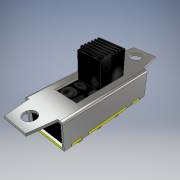
# Autodesk Inventor part: Switch-T220
Saved by Autodesk Inventor 2018 (Build 220112000, 112)
## iProperties
Created: 2021-02-15
Part Number: Switch-T220
Material: Všeobecné
Document SubType Name: Modeling
Designer: Jozko Mrkvicka
Density: 1 g/cm^3
Appearance: Výchozí
Author: Jozko Mrkvicka
Autodesk Inventor part; units mm, degrees
ref_plane "YZ Plane" through (0, 0, 0) normal (1, 0, 0) x (0, 1, 0)
ref_plane "XZ Plane" through (0, 0, 0) normal (0, 1, 0) x (-1, 0, 0)
sketch "Náčrt1" plane through (0, 0, 0) normal (0, 1, 0) x (-1, 0, 0)
  line L0 (-3.175, 18.0975) -> (3.175, 18.0975)
  line L1 (5.3975, 12.065) -> (5.3975, -12.065)
  line L2 (3.175, -18.0975) -> (-3.175, -18.0975)
  line L3 (-5.3975, -12.065) -> (-5.3975, 12.065)
  line L4 (3.175, 18.0975) -> (4.1275, 12.065)
  line L5 (-4.1275, 12.065) -> (-3.175, 18.0975)
  line L6 (-4.1275, -12.065) -> (-3.175, -18.0975)
  line L7 (4.1275, -12.065) -> (3.175, -18.0975)
  circle A0 centre (0, 14.9225) radius 1.5875
  circle A1 centre (0, -14.9225) radius 1.5875
  line L8 (-5.3975, 12.065) -> (-4.1275, 12.065)
  line L9 (4.1275, 12.065) -> (5.3975, 12.065)
  line L10 (5.3975, -12.065) -> (4.1275, -12.065)
  line L11 (-4.1275, -12.065) -> (-5.3975, -12.065)
  line L12 (-3.175, 6.6675) -> (3.175, 6.6675)
  line L13 (3.175, 6.6675) -> (3.175, -6.6675)
  line L14 (3.175, -6.6675) -> (-3.175, -6.6675)
  line L15 (-3.175, -6.6675) -> (-3.175, 6.6675)
  line L16 (-3.175, 6.6675) -> (3.175, -6.6675) construction
  line L17 (3.175, 6.6675) -> (-3.175, -6.6675) construction
  point P0 (0, 0)
  dimension "d7" = 6.35
  dimension "d8" = 13.335
  constraints: 36 end point, 8 parallel, 4 horizontal, 2 centre point, 2 midpoint, 2 perpendicular
  measures "d7" distance of L13.end L14.end
  measures "d8" distance of L12.end L13.end
extrude "Vysunutí1" add sketch "Náčrt1" along normal blind 0.635
sketch "Náčrt2" plane through (0, 0, 0) normal (0, -1, 0) x (1, 0, 0)
  line L0 (5.3975, 12.065) -> (4.1275, 12.065) projected
  line L1 (-5.3975, -12.065) -> (-5.3975, 12.065) projected
  line L2 (5.3975, 12.065) -> (-5.3975, 12.065)
  line L3 (-5.3975, 12.065) -> (-5.3975, -12.065)
  line L4 (-5.3975, -12.065) -> (5.3975, -12.065)
  line L5 (5.3975, -12.065) -> (5.3975, 12.065)
  constraints: 8 end point, 2 parallel, 1 horizontal, 1 perpendicular
extrude "Vysunutí2" add sketch "Náčrt2" along normal blind 6.35
sketch "Náčrt3" plane through (0, 0, 0) normal (0, 1, 0) x (1, 0, 0)
  line L0 (3.175, 6.6675) -> (3.175, -6.6675) projected
  line L1 (-3.175, -6.6675) -> (3.175, -6.6675)
  line L2 (3.175, -6.6675) -> (3.175, 0.3175)
  line L3 (3.175, 0.3175) -> (-3.175, 0.3175)
  line L4 (-3.175, 0.3175) -> (-3.175, -6.6675)
  point P0 (0, 0)
  dimension "d13" = 6.985
  constraints: 8 end point, 2 parallel, 1 horizontal, 1 perpendicular, 1 point on line
  measures "d13" distance of L2.end L1.end
extrude "Vysunutí3" add sketch "Náčrt3" along normal blind 6.985
sketch "Náčrt4" plane through (3.175, 0.635, -0.3175) normal (1, 0, 0) x (0, 0, -1)
  line L0 (-6.985, 6.35) -> (0, 6.35) projected
  line L1 (-6.223, 6.35) -> (-5.588, 6.35)
  line L2 (-5.588, 6.35) -> (-5.588, 6.6675)
  line L3 (-6.223, 6.6675) -> (-6.223, 6.35)
  arc A0 (-5.588, 6.6675) -> (-6.223, 6.6675) centre (-5.9055, 6.6675) ccw
  line L4 (-5.2705, 6.35) -> (-4.6355, 6.35)
  line L5 (-4.6355, 6.35) -> (-4.6355, 6.6675)
  line L6 (-5.2705, 6.6675) -> (-5.2705, 6.35)
  arc A1 (-4.6355, 6.6675) -> (-5.2705, 6.6675) centre (-4.953, 6.6675) ccw
  line L7 (-4.318, 6.35) -> (-3.683, 6.35)
  line L8 (-3.683, 6.35) -> (-3.683, 6.6675)
  line L9 (-4.318, 6.6675) -> (-4.318, 6.35)
  arc A2 (-3.683, 6.6675) -> (-4.318, 6.6675) centre (-4.0005, 6.6675) ccw
  line L10 (-3.3655, 6.35) -> (-2.7305, 6.35)
  line L11 (-2.7305, 6.35) -> (-2.7305, 6.6675)
  line L12 (-3.3655, 6.6675) -> (-3.3655, 6.35)
  arc A3 (-2.7305, 6.6675) -> (-3.3655, 6.6675) centre (-3.048, 6.6675) ccw
  line L13 (-2.413, 6.35) -> (-1.778, 6.35)
  line L14 (-1.778, 6.35) -> (-1.778, 6.6675)
  line L15 (-2.413, 6.6675) -> (-2.413, 6.35)
  arc A4 (-1.778, 6.6675) -> (-2.413, 6.6675) centre (-2.0955, 6.6675) ccw
  line L16 (-1.4605, 6.35) -> (-0.8255, 6.35)
  line L17 (-0.8255, 6.35) -> (-0.8255, 6.6675)
  line L18 (-1.4605, 6.6675) -> (-1.4605, 6.35)
  arc A5 (-0.8255, 6.6675) -> (-1.4605, 6.6675) centre (-1.143, 6.6675) ccw
  point P0 (-0.3175, -0.635)
  dimension "d28" = 0.9525
  constraints: 36 end point, 12 point on circle, 6 centre point, 2 horizontal, 1 parallel, 1 perpendicular, 1 point on line, 45 other
  measures "d28" distance of L1.start L4.start
extrude "Vysunutí4" add sketch "Náčrt4" against normal up to surface (6.35 mm away)
fillet "Zaoblení1" radius 0.635 2 edges at (5.3975, 0.635, 0) (-5.3975, 0.635, 0)
sketch "Náčrt5" plane through (0, -6.35, 0) normal (0, -1, 0) x (1, 0, 0)
  line L0 (5.3975, 12.065) -> (4.7625, 12.065)
  line L1 (4.7625, 12.065) -> (4.7625, 10.16)
  line L2 (4.7625, 10.16) -> (5.3975, 10.16)
  line L3 (5.3975, 10.16) -> (5.3975, 12.065)
  line L4 (5.3975, -12.065) -> (4.7625, -12.065)
  line L5 (4.7625, -12.065) -> (4.7625, -10.16)
  line L6 (4.7625, -10.16) -> (5.3975, -10.16)
  line L7 (5.3975, -10.16) -> (5.3975, -12.065)
  line L8 (-5.3975, -12.065) -> (-4.7625, -12.065)
  line L9 (-4.7625, -12.065) -> (-4.7625, -10.16)
  line L10 (-4.7625, -10.16) -> (-5.3975, -10.16)
  line L11 (-5.3975, -10.16) -> (-5.3975, -12.065)
  line L12 (-5.3975, 12.065) -> (-4.7625, 12.065)
  line L13 (-4.7625, 12.065) -> (-4.7625, 10.16)
  line L14 (-4.7625, 10.16) -> (-5.3975, 10.16)
  line L15 (-5.3975, 10.16) -> (-5.3975, 12.065)
  line L16 (4.7625, -7.62) -> (5.3975, -7.62)
  line L17 (5.3975, -7.62) -> (5.3975, -5.715)
  line L18 (5.3975, -5.715) -> (4.7625, -5.715)
  line L19 (4.7625, -5.715) -> (4.7625, -7.62)
  line L20 (-4.7625, 7.62) -> (-5.3975, 7.62)
  line L21 (-5.3975, 7.62) -> (-5.3975, 5.715)
  line L22 (-5.3975, 5.715) -> (-4.7625, 5.715)
  line L23 (-4.7625, 5.715) -> (-4.7625, 7.62)
  line L24 (4.7625, 7.62) -> (5.3975, 7.62)
  line L25 (5.3975, 7.62) -> (5.3975, 5.715)
  line L26 (5.3975, 5.715) -> (4.7625, 5.715)
  line L27 (4.7625, 5.715) -> (4.7625, 7.62)
  line L28 (-4.7625, -7.62) -> (-5.3975, -7.62)
  line L29 (-5.3975, -7.62) -> (-5.3975, -5.715)
  line L30 (-5.3975, -5.715) -> (-4.7625, -5.715)
  line L31 (-4.7625, -5.715) -> (-4.7625, -7.62)
  line L32 (5.3975, 12.065) -> (-5.3975, 12.065)
  line L33 (-5.3975, 12.065) -> (-5.3975, -12.065)
  line L34 (-5.3975, -12.065) -> (5.3975, -12.065)
  line L35 (5.3975, -12.065) -> (5.3975, 12.065)
  point P0 (0, 0)
  constraints: 72 end point, 18 parallel, 9 horizontal, 9 perpendicular, 6 point on line
extrude "Vysunutí5" cut sketch "Náčrt5" against normal blind 0.635 contours L3 L2 L1 L0 | L13 L14 L15 L12 | L25 L26 L27 L24 | L17 L16 L19 L18 | L20 L23 L22 L21 | L7 L4 L5 L6 | L30 L31 L28 L29 | L10 L9 L8 L11
ref_plane "Pracovní rovina1" through (4.7625, -5.715, -12.065) normal (0, -1, 0) x (1, 0, 0)
split_face "Rozdělit1"
sketch "Náčrt6" plane through (0, -5.715, 0) normal (0, -1, 0) x (1, 0, 0)
  line L0 (-5.3975, -12.065) -> (-4.8809, -12.065)
  line L1 (-4.8809, -12.065) -> (-4.8809, -10.287)
  line L2 (-4.8809, -10.287) -> (-5.3975, -10.287)
  line L3 (-5.3975, -10.287) -> (-5.3975, -12.065)
  line L4 (-5.3975, 10.287) -> (-4.8809, 10.287)
  line L5 (-4.8809, 10.287) -> (-4.8809, 12.065)
  line L6 (-4.8809, 12.065) -> (-5.3975, 12.065)
  line L7 (-5.3975, 12.065) -> (-5.3975, 10.287)
  line L8 (5.3975, 12.065) -> (4.8872, 12.065)
  line L9 (4.8872, 12.065) -> (4.8872, 10.287)
  line L10 (4.8872, 10.287) -> (5.3975, 10.287)
  line L11 (5.3975, 10.287) -> (5.3975, 12.065)
  line L12 (5.3975, -12.065) -> (4.7625, -12.065)
  line L13 (5.3975, -10.287) -> (4.8872, -10.287)
  line L14 (4.8872, -10.287) -> (4.8872, -12.065)
  line L15 (4.8872, -12.065) -> (5.3975, -12.065)
  line L16 (5.3975, -12.065) -> (5.3975, -10.287)
  point P0 (-5.3975, 5.715)
  point P1 (5.3975, 7.62)
  point P2 (5.3975, -5.715)
  dimension "d46" = 1.778
  dimension "d48" = 1.778
  dimension "d49" = 1.778
  dimension "d50" = 1.778
  constraints: 34 end point, 2 parallel, 1 horizontal, 1 perpendicular, 1 point on line, 3 other
  measures "d46" distance between parallel lines of L0 L2
  measures "d48" distance between parallel lines of L4 L6
  measures "d49" distance of L15.end L13.start
  measures "d50" distance of L10.end L8.start
extrude "Vysunutí6" add sketch "Náčrt6" along normal blind 0.635
sketch "Náčrt7" plane through (0, -5.715, 0) normal (0, -1, 0) x (1, 0, 0)
  line L0 (-4.8895, -7.5565) -> (-5.3975, -7.5565)
  line L1 (-5.3975, -7.5565) -> (-5.3975, -5.7785)
  line L2 (-5.3975, -5.7785) -> (-4.8895, -5.7785)
  line L3 (-4.8895, -5.7785) -> (-4.8895, -7.5565)
  line L4 (-4.8895, -7.5565) -> (-5.3975, -5.7785) construction
  line L5 (-5.3975, -7.5565) -> (-4.8895, -5.7785) construction
  line L6 (-4.8895, 5.7785) -> (-5.3975, 5.7785)
  line L7 (-5.3975, 5.7785) -> (-5.3975, 7.5565)
  line L8 (-5.3975, 7.5565) -> (-4.8895, 7.5565)
  line L9 (-4.8895, 7.5565) -> (-4.8895, 5.7785)
  line L10 (-4.8895, 5.7785) -> (-5.3975, 7.5565) construction
  line L11 (-5.3975, 5.7785) -> (-4.8895, 7.5565) construction
  line L12 (5.3975, -7.5565) -> (4.8895, -7.5565)
  line L13 (4.8895, -7.5565) -> (4.8895, -5.7785)
  line L14 (4.8895, -5.7785) -> (5.3975, -5.7785)
  line L15 (5.3975, -5.7785) -> (5.3975, -7.5565)
  line L16 (5.3975, -7.5565) -> (4.8895, -5.7785) construction
  line L17 (4.8895, -7.5565) -> (5.3975, -5.7785) construction
  line L18 (5.3975, 5.7785) -> (4.8895, 5.7785)
  line L19 (4.8895, 5.7785) -> (4.8895, 7.5565)
  line L20 (4.8895, 7.5565) -> (5.3975, 7.5565)
  line L21 (5.3975, 7.5565) -> (5.3975, 5.7785)
  line L22 (5.3975, 5.7785) -> (4.8895, 7.5565) construction
  line L23 (4.8895, 5.7785) -> (5.3975, 7.5565) construction
  point P0 (0, 0)
  point P1 (-5.1435, -6.6675)
  point P2 (-5.1435, 6.6675)
  point P3 (5.1435, -6.6675)
  point P4 (5.1435, 6.6675)
  dimension "d53" = 1.778
  dimension "d54" = 1.778
  dimension "d55" = 1.778
  dimension "d56" = 1.778
  dimension "d57" = 0.508
  dimension "d59" = 0.508
  dimension "d60" = 0.508
  dimension "d61" = 0.508
  constraints: 48 end point, 8 midpoint, 8 parallel, 4 horizontal, 4 perpendicular, 4 other
  measures "d53" distance of L0.end L1.end
  measures "d54" distance of L6.end L7.end
  measures "d55" distance of L12.end L13.end
  measures "d56" distance of L18.end L19.end
  measures "d57" distance of L13.end L14.end
  measures "d59" distance of L19.end L20.end
  measures "d60" distance of L6.start L6.end
  measures "d61" distance of L0.start L0.end
extrude "Vysunutí7" add sketch "Náčrt7" along normal blind 0.635
sketch "Náčrt8" plane through (-4.7625, -5.715, 12.065) normal (0, 0, 1) x (1, 0, 0)
  line L0 (-0.1184, 0) -> (9.6497, 0)
  line L1 (9.6497, 0) -> (9.6497, 5.715)
  line L2 (9.6497, 5.715) -> (-0.1184, 5.715)
  line L3 (-0.1184, 5.715) -> (-0.1184, 0)
  point P0 (4.7625, 5.715)
  constraints: 8 end point, 2 parallel, 1 horizontal, 1 perpendicular
extrude "Vysunutí8" cut sketch "Náčrt8" against normal blind 0.635
sketch "Náčrt9" plane through (4.7625, -5.715, -12.065) normal (0, 0, -1) x (-1, 0, 0)
  line L0 (-0.1247, 0) -> (0, 0) projected
  line L1 (-0.1247, 5.715) -> (-0.1247, 0) projected
  line L2 (9.6434, 5.715) -> (-0.1247, 5.715) projected
  line L3 (9.6434, 0) -> (9.6434, 5.715) projected
  line L4 (9.525, 0) -> (9.6434, 0) projected
  line L5 (0, 0) -> (9.525, 0) projected
  point P0 (4.7625, 5.715)
extrude "Vysunutí9" cut sketch "Náčrt9" against normal blind 0.635
sketch "Náčrt10" plane through (0, -6.35, 0) normal (0, -1, 0) x (1, 0, 0)
  line L0 (-4.7625, 7.62) -> (-4.7625, 5.715)
  line L1 (-4.7625, -5.715) -> (-4.7625, -7.62)
  line L2 (5.3975, -5.715) -> (5.3975, 5.715) projected
  line L3 (5.3975, 5.715) -> (4.7625, 5.715) projected
  line L4 (5.3975, -5.715) -> (5.3975, 0)
  line L5 (2.2225, 6.6675) -> (2.8575, 6.6675)
  line L6 (2.8575, 6.6675) -> (2.8575, 4.7625)
  line L7 (2.8575, 4.7625) -> (2.2225, 4.7625)
  line L8 (2.2225, 4.7625) -> (2.2225, 6.6675)
  line L9 (2.2225, 0.9525) -> (2.8575, 0.9525)
  line L10 (2.8575, 0.9525) -> (2.8575, -0.9525)
  line L11 (2.2225, -0.9525) -> (2.2225, 0.9525)
  line L12 (2.8575, -0.9525) -> (2.2225, -0.9525)
  line L13 (2.2225, -4.7625) -> (2.8575, -4.7625)
  line L14 (2.8575, -4.7625) -> (2.8575, -6.6675)
  line L15 (2.2225, -6.6675) -> (2.2225, -4.7625)
  line L16 (2.8575, -6.6675) -> (2.2225, -6.6675)
  line L17 (-2.8575, 6.6675) -> (-2.2225, 6.6675)
  line L18 (-2.2225, 6.6675) -> (-2.2225, 4.7625)
  line L19 (-2.8575, 4.7625) -> (-2.8575, 6.6675)
  line L20 (-2.2225, 4.7625) -> (-2.8575, 4.7625)
  line L21 (-2.8575, 0.9525) -> (-2.2225, 0.9525)
  line L22 (-2.2225, 0.9525) -> (-2.2225, -0.9525)
  line L23 (-2.8575, -0.9525) -> (-2.8575, 0.9525)
  line L24 (-2.2225, -0.9525) -> (-2.8575, -0.9525)
  line L25 (-2.8575, -4.7625) -> (-2.2225, -4.7625)
  line L26 (-2.2225, -4.7625) -> (-2.2225, -6.6675)
  line L27 (-2.8575, -6.6675) -> (-2.8575, -4.7625)
  line L28 (-2.2225, -6.6675) -> (-2.8575, -6.6675)
  dimension "d83" = 5.715
  dimension "d86" = 5.08
  constraints: 54 end point, 1 horizontal, 1 midpoint, 1 vertical, 40 other
  measures "d83" distance of L5.end L9.end
  measures "d86" distance of L5.end L17.end
extrude "Vysunutí10" add sketch "Náčrt10" along normal blind 3.81
sketch "Náčrt11" plane through (2.8575, -6.35, 6.6675) normal (1, 0, 0) x (0, 0, -1)
  line L0 (0, -3.81) -> (1.905, -3.81) projected
  line L1 (1.905, 0) -> (1.905, -3.81) projected
  circle A0 centre (0.9525, -2.8575) radius 0.635
  circle A1 centre (6.6675, -2.8575) radius 0.635
  circle A2 centre (12.3825, -2.8575) radius 0.635
  point P0 (6.6675, 6.35)
  dimension "d91" = 1.27
  dimension "d92" = 1.27
  dimension "d93" = 1.27
  constraints: 3 centre point
  measures "d91" diameter of A0
  measures "d92" diameter of A1
  measures "d93" diameter of A2
extrude "Vysunutí11" cut sketch "Náčrt11" against normal up to surface (5.715 mm away)
fillet "Zaoblení2" radius 0.9525 12 edges at (2.54, -10.16, 6.6675) (2.54, -10.16, 4.7625) (-2.54, -10.16, 6.6675) (-2.54, -10.16, 4.7625) (-2.54, -10.16, 0.9525) (-2.54, -10.16, -0.9525) (-2.54, -10.16, -4.7625) (-2.54, -10.16, -6.6675) (2.54, -10.16, 0.9525) (2.54, -10.16, -0.9525) (2.54, -10.16, -4.7625) (2.54, -10.16, -6.6675)
